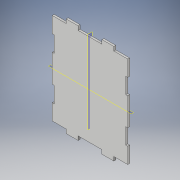
# Autodesk Inventor part: rev1 small wall
Saved by Autodesk Inventor 2017 (Build 210142000, 142)
## iProperties
Created: 2019-05-03
Part Number: rev1 small wall
Material: Generic
Document SubType Name: Modeling
Designer: Roman
Density: 1 g/cm^3
Appearance: Default
Author: Roman
Autodesk Inventor part; units mm, degrees
ref_plane "YZ Plane" through (0, 0, 0) normal (1, 0, 0) x (0, 1, 0)
ref_plane "XZ Plane" through (0, 0, 0) normal (0, 1, 0) x (-1, 0, 0)
ref_plane "XY Plane" through (0, 0, 0) normal (0, 0, 1) x (1, 0, 0)
sketch "Sketch1" plane through (0, 0, 0) normal (0, 0, 1) x (1, 0, 0)
  line L0 (0, 0) -> (965.2, 0)
  line L1 (965.2, 0) -> (965.2, -1168.4)
  line L2 (965.2, -1168.4) -> (0, -1168.4)
  line L3 (0, -1168.4) -> (0, 0)
  dimension "d0" = 965.2
  dimension "d1" = 1168.4
  constraints: 8 end point, 2 parallel, 1 horizontal, 1 perpendicular
  measures "d0" distance of L1.end L2.end
  measures "d1" distance of L0.end L1.end
extrude "Extrusion1" add sketch "Sketch1" along normal blind 25.4
sketch "Sketch2" plane through (0, -1168.4, 0) normal (0, -1, 0) x (1, 0, 0)
  line L0 (965.2, 25.4) -> (0, 25.4) projected
  line L1 (0, 0) -> (965.2, 0) projected
  line L2 (177.8, 25.4) -> (330.2, 25.4)
  line L3 (330.2, 25.4) -> (330.2, 0)
  line L4 (330.2, 0) -> (177.8, 0)
  line L5 (177.8, 0) -> (177.8, 25.4)
  line L6 (177.8, 12.7) -> (330.2, 12.7)
  line L7 (635, 25.4) -> (787.4, 25.4)
  line L8 (787.4, 25.4) -> (787.4, 0)
  line L9 (787.4, 0) -> (635, 0)
  line L10 (635, 0) -> (635, 25.4)
  line L11 (635, 12.7) -> (787.4, 12.7)
  line L12 (787.4, 12.7) -> (965.2, 12.7)
  line L13 (965.2, 0) -> (965.2, 25.4) projected
  line L14 (965.2, 0) -> (0, 0) projected
  line L15 (965.2, 0) -> (965.2, 25.4) projected
  line L16 (0, 25.4) -> (965.2, 25.4) projected
  line L17 (0, 0) -> (0, 25.4) projected
  line L18 (177.8, 12.7) -> (0, 12.7)
  line L19 (0, 0) -> (0, 25.4) projected
  dimension "d4" = 152.4
  dimension "d5" = 177.8
  constraints: 24 end point, 6 midpoint, 4 parallel, 4 point on line, 2 collinear, 2 horizontal, 2 perpendicular
  measures "d4" distance of L6.start L6.end
  measures "d5" distance of L6.start L18.end
extrude "Extrusion2" add sketch "Sketch2" along normal blind 50.8 contours L8 L11 L10 L0 | L8 L1 L10 L11 | L3 L6 L5 L0 | L3 L1 L5 L6
sketch "Sketch3" plane through (0, -1168.4, 0) normal (-1, 0, 0) x (0, 0, 1)
  line L0 (0, 0) -> (0, 1168.4) projected
  line L1 (0, 0) -> (25.4, 0) projected
  line L2 (25.4, 1168.4) -> (25.4, 0) projected
  line L3 (0, 1168.4) -> (25.4, 1168.4) projected
  line L4 (25.4, 1168.4) -> (25.4, 0) projected
  line L5 (0, 203.2) -> (25.4, 203.2)
  line L6 (25.4, 203.2) -> (25.4, 406.4)
  line L7 (25.4, 406.4) -> (0, 406.4)
  line L8 (0, 406.4) -> (0, 203.2)
  line L9 (0, 0) -> (0, 1168.4) projected
  line L10 (0, 965.2) -> (25.4, 965.2)
  line L11 (25.4, 965.2) -> (25.4, 762)
  line L12 (25.4, 762) -> (0, 762)
  line L13 (0, 762) -> (0, 965.2)
  dimension "d8" = 203.2
  dimension "d9" = 203.2
  dimension "d12" = 355.6
  dimension "d13" = 203.2
  constraints: 16 end point, 4 parallel, 4 point on line, 2 horizontal, 2 perpendicular
  measures "d8" distance between parallel lines of L1 L5
  measures "d9" distance between parallel lines of L5 L7
  measures "d12" distance between parallel lines of L7 L12
  measures "d13" distance between parallel lines of L12 L10
extrude "Extrusion3" cut sketch "Sketch3" against normal blind 25.4 contours L0 L7 L2 L5 | L0 L10 L2 L12
ref_plane "Work Plane1" through (482.6, 0, 0) normal (-1, 0, 0) x (0, 0, 1)
mirror "Mirror1" about plane through (482.6, 0, 0) normal (-1, 0, 0) of "Extrusion3"
ref_plane "Work Plane2" through (330.2, -584.2, 0) normal (0, -1, 0) x (1, 0, 0)
mirror "Mirror2" about plane through (330.2, -584.2, 0) normal (0, -1, 0) of "Extrusion2"
body "Solid1"
